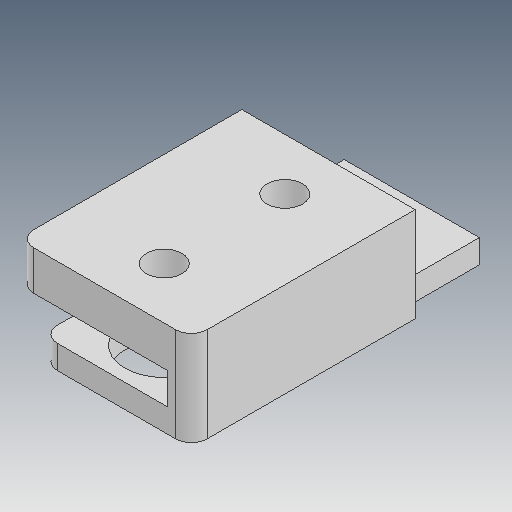
# Autodesk Inventor part: imu_housing_op
Saved by Autodesk Inventor 2025.2 (Build 292293000, 293)
## iProperties
Created: 2025-02-13
Part Number: imu_housing_op
Material: Generic
Document SubType Name: Modeling
Designer: Alex
Density: 1 g/cm^3
Appearance: Default
Author: Alex
Autodesk Inventor part; units mm, degrees
ref_plane "YZ Plane" through (0, 0, 0) normal (1, 0, 0) x (0, 1, 0)
ref_plane "XZ Plane" through (0, 0, 0) normal (0, 1, 0) x (-1, 0, 0)
ref_plane "XY Plane" through (0, 0, 0) normal (0, 0, 1) x (1, 0, 0)
sketch "Sketch1" plane through (0, 0, 0) normal (0, 0, 1) x (1, 0, 0)
  line L0 (0, 0) -> (15, 0)
  line L1 (15, 0) -> (15, 3)
  line L2 (15, 3) -> (0, 3)
  line L3 (0, 3) -> (0, 0)
  line L4 (15, 0) -> (12, 0)
  line L5 (12, 0) -> (12, 7)
  line L6 (12, 7) -> (15, 7)
  line L7 (15, 7) -> (15, 0)
  line L8 (15, 7) -> (-3, 7)
  line L9 (-3, 7) -> (-3, 12)
  line L10 (-3, 12) -> (15, 12)
  line L11 (15, 12) -> (15, 7)
  line L12 (12, 3) -> (0, 3) construction
  line L13 (6, 3) -> (6, 0) construction
  dimension "d0" = 3
  dimension "d1" = 3
  dimension "d2" = 5
  dimension "d4" = 12
  dimension "d5" = 18
  dimension "d7" = 6
  constraints: 28 end point, 6 parallel, 4 perpendicular, 3 horizontal, 3 point on line, 1 collinear, 1 midpoint
  measures "d0" distance between parallel lines of L0 L2
  measures "d1" distance between parallel lines of L7 L5
  measures "d2" distance between parallel lines of L8 L10
  measures "d4" distance between parallel lines of L0 L10
  measures "d5" distance of L9.end L10.end
  measures "d7" distance between parallel lines of L5 L13
extrude "Extrusion1" add sketch "Sketch1" along normal blind 28 and the other way blind 0.4
sketch "Sketch2" plane through (0, 3, -0.4) normal (0, 1, 0) x (1, 0, 0)
  circle A0 centre (5, -6.55) radius 1.45
  circle A1 centre (5, -21.85) radius 1.45
  line L0 (12, 0) -> (12, -28.4) projected
  line L1 (15, -28.4) -> (15, 0) projected
  line L2 (15, 0) -> (15, -28.4) projected
  line L3 (5, -6.55) -> (5, -21.85) construction
  line L4 (5, -14.2) -> (12, -14.2) construction
  circle A2 centre (5, -21.85) radius 5
  circle A3 centre (5, -6.55) radius 5
  point P0 (0, -0.4)
  dimension "d10" = 10
  dimension "d11" = 2.9
  dimension "d12" = 15.3
  dimension "d13" = 10
  dimension "d14" = 10
  constraints: 4 centre point, 4 end point, 2 coincident, 2 midpoint, 1 equal radius, 1 perpendicular, 1 vertical, 1 vertical alignment
  measures "d10" distance from line of L1 L3.end
  measures "d11" diameter of A1
  measures "d12" distance of L3.start L3.end
  measures "d13" diameter of A2
  measures "d14" diameter of A3
extrude "Extrusion2" cut sketch "Sketch2" against normal up to surface (3 mm away) contours A0 | A1 | A2 | A3
sketch "Sketch3" plane through (-3, 12, -0.4) normal (0, 1, 0) x (1, 0, 0)
  circle A0 centre (8, -21.85) radius 4 construction
  circle A1 centre (8, -6.55) radius 4 construction
  circle A2 centre (8, -6.55) radius 5.5
  circle A3 centre (8, -21.85) radius 5.5
  circle A4 centre (8, -6.55) radius 2.25
  circle A5 centre (8, -21.85) radius 2.25
  point P0 (3, -0.4)
  dimension "d21" = 1.5
  dimension "d22" = 1.5
  dimension "d50" = 4.5
  constraints: 4 centre point, 2 coincident, 1 equal radius
  measures "d21" radial gap between concentric circles of A1 A2
  measures "d22" radial gap between concentric circles of A0 A3
  measures "d50" diameter of A4
extrude "Extrusion5" cut sketch "Sketch3" against normal up to surface (5 mm away) contours A4 | A5
sketch "Sketch4" plane through (0, 0, -0.4) normal (-1, 0, 0) x (0, 0, 1)
  line L0 (0, 0) -> (6.55, 0) projected
  line L1 (28.4, 3) -> (28.4, 0) projected
  line L2 (0, 3) -> (6.55, 3) projected
  line L3 (0, 0) -> (0, 3) projected
  line L4 (6.55, 3) -> (6.55, 0) projected
  line L5 (6.55, 0) -> (21.85, 0) projected
  line L6 (21.85, 3) -> (21.85, 0) projected
  line L7 (6.55, 3) -> (21.85, 3) projected
  line L8 (21.85, 0) -> (28.4, 0) projected
  line L9 (21.85, 3) -> (28.4, 3) projected
  line L10 (0, 3) -> (28.4, 3)
  line L11 (28.4, 3) -> (28.4, 0)
  line L12 (28.4, 0) -> (0, 0)
  line L13 (0, 0) -> (0, 3)
  point P0 (0.4, 0)
  constraints: 8 end point, 2 parallel, 1 horizontal, 1 perpendicular
extrude "Extrusion6" add sketch "Sketch4" along normal blind 4 from surface at 0
sketch "Sketch8" plane through (-3, 7, -0.4) normal (-1, 0, 0) x (0, 0, 1)
  line L0 (0, 0) -> (0, 5) projected
  line L1 (0, 0) -> (28.4, 0) projected
  line L2 (28.4, 5) -> (28.4, 0) projected
  line L3 (0, 5) -> (28.4, 5) projected
  point P0 (0.4, -7)
extrude "Extrusion10" add sketch "Sketch8" along normal blind 4
extrude "Extrusion11" add sketch "Sketch8" along normal blind 4
sketch "Sketch10" plane through (0, 0, -0.4) normal (0, 0, -1) x (-1, 0, 0)
  line L0 (4, 0) -> (-15, 0) projected
  line L1 (4, 3) -> (-13.15, 3)
  line L2 (-13.15, 3) -> (-13.15, 0)
  line L3 (-13.15, 0) -> (4, 0)
  line L4 (4, 0) -> (4, 3)
  dimension "d51" = 17.15
  constraints: 8 end point, 2 parallel, 1 horizontal, 1 perpendicular, 1 point on line
  measures "d51" distance between parallel lines of L4 L2
extrude "Extrusion13" add sketch "Sketch10" along normal blind 10
sketch "Sketch11" plane through (-4, 0, 28) normal (0, -1, 0) x (1, 0, 0)
  line L0 (19, -28.4) -> (19, 0) construction
  circle A0 centre (8.55, -33.55) radius 1.65
  circle A1 centre (9, -6.55) radius 5 projected
  circle A2 centre (9, -21.85) radius 5 projected
  line L1 (0, 0) -> (0, -38.4) projected
  line L2 (0, 0) -> (19, 0) projected
  line L3 (19, -28.4) -> (17.15, -28.4) projected
  line L4 (17.15, -38.4) -> (0, -38.4) projected
  line L5 (17.15, -28.4) -> (17.15, -38.4) projected
  point P0 (4, -28)
  point P1 (8.55, -38.4)
  point P2 (18.075, -28.4)
  dimension "d45" = 3.3
  dimension "d52" = 5.15
  dimension "d53" = 8.6
  constraints: 1 centre point, 1 midpoint, 1 vertical alignment
  measures "d45" diameter of A0
  measures "d52" vertical distance of point (18.075, -28.4) A0.centre
  measures "d53" distance from line of L5 A0.centre
extrude "Extrusion14" cut sketch "Sketch11" against normal up to next contours A0
fillet "Fillet1" radius 2 3 edges at (15, 6, 28) (-4, 1.5, 28) (-7, 9.5, 28)
body "Solid1"
